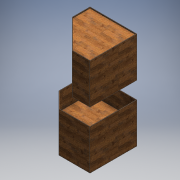
# Autodesk Inventor part: esquinero
Saved by Autodesk Inventor 2016 (Build 200138000, 138)
## iProperties
Created: 2015-11-25
Part Number: esquinero
Material: Generic
Document SubType Name: Modeling
Designer: Daniela
Density: 1 g/cm^3
Appearance: White
Author: Daniela
Autodesk Inventor part; units mm, degrees
ref_plane "YZ Plane" through (0, 0, 0) normal (1, 0, 0) x (0, 1, 0)
ref_plane "XZ Plane" through (0, 0, 0) normal (0, 1, 0) x (-1, 0, 0)
ref_plane "XY Plane" through (0, 0, 0) normal (0, 0, 1) x (1, 0, 0)
sketch "Sketch2" plane through (0, 0, 0) normal (0, 0, 1) x (1, 0, 0)
  line L0 (0, 0) -> (1050, 0) construction
  line L1 (1050, 0) -> (1050, 1050) construction
  line L2 (1050, 1050) -> (0, 1050) construction
  line L3 (0, 1050) -> (0, 0) construction
  line L4 (350, 0) -> (0, 350)
  line L5 (0, 350) -> (0, 1050)
  line L6 (0, 1050) -> (1050, 1050)
  line L7 (1050, 1050) -> (1050, 0)
  line L8 (1050, 0) -> (350, 0)
  dimension "d6" = 45
  dimension "profundidad" = 700
  dimension "d8" = 350
  constraints: 18 end point, 4 collinear, 2 parallel, 2 perpendicular, 2 point on line, 1 horizontal
  measures "d6" angle of L4 L0
  measures "profundidad" distance from line of L2 L4.end
  measures "d8" distance of L0.start L4.end
extrude "Extrusion1" add sketch "Sketch2" along normal blind 10
ref_plane "Work Plane1" through (0, 0, -80) normal (0, 0, -1) x (-1, 0, 0)
sketch "Sketch4" plane through (0, 0, -80) normal (0, 0, -1) x (-1, 0, 0)
  line L0 (-1050, 1050) -> (0, 1050) projected
  line L1 (-1050, 0) -> (-1050, 1050) projected
  line L2 (-350, 0) -> (-1050, 0) projected
  line L3 (0, 350) -> (-350, 0) projected
  line L4 (0, 1050) -> (0, 350) projected
  line L5 (-1040, 1040) -> (-10, 1040)
  line L6 (-10, 1040) -> (-10, 354.1421)
  line L7 (-10, 354.1421) -> (-354.1421, 10)
  line L8 (-354.1421, 10) -> (-1040, 10)
  line L9 (-1040, 10) -> (-1040, 1040)
  point P0 (0, 0)
  dimension "d12" = 10
  constraints: 10 end point, 4 other
  measures "d12" distance between parallel lines of L9 L1
extrude "Extrusion2" add sketch "Sketch4" against normal blind 900
sketch "Sketch5" plane through (350, 0, 820) normal (-0.7071068, -0.7071068, 0) x (-0.7071068, 0.7071068, 0)
  line L0 (0, 900) -> (0, 0) construction
  line L1 (494.9747, 900) -> (494.9747, 0) construction
  line L2 (494.9747, 0) -> (0, 0) construction
  line L3 (490.8326, 810) -> (4.1421, 810) construction
  line L4 (464.9747, 30) -> (34.1421, 30)
  line L5 (34.1421, 30) -> (34.1421, 810)
  line L6 (34.1421, 810) -> (464.9747, 810)
  line L7 (464.9747, 810) -> (464.9747, 30)
  line L8 (4.1421, 810) -> (4.1421, 0) projected
  point P0 (247.4874, 820)
  dimension "d15" = 30
  dimension "d16" = 30
  dimension "d17" = 30
  dimension "d18" = 0
  constraints: 8 end point, 2 parallel, 1 horizontal, 1 perpendicular
  measures "d15" distance between parallel lines of L2 L4
  measures "d16" distance between parallel lines of L1 L7
  measures "d17" distance between parallel lines of L8 L5
  measures "d18" distance between parallel lines of L3 L6
extrude "Extrusion3" cut sketch "Sketch5" against normal up to next
ref_plane "Work Plane2" through (0, 0, 1200) normal (0, 0, 1) x (1, 0, 0)
sketch "Sketch12" plane through (0, 0, 1200) normal (0, 0, 1) x (1, 0, 0)
  line L0 (1050, 1050) -> (0, 1050) projected
  line L1 (0, 1050) -> (0, 350) construction
  line L2 (0, 350) -> (350, 0) construction
  line L3 (350, 0) -> (1050, 0) construction
  line L4 (1050, 0) -> (1050, 1050) projected
  line L5 (0, 650) -> (650, 0)
  line L6 (0, 650) -> (0, 1050)
  line L7 (650, 0) -> (1050, 0)
  point P0 (0, 0)
  dimension "d32" = 400
  constraints: 6 end point, 2 collinear, 2 point on line, 1 parallel
  measures "d32" distance from line of L0 L5.start
extrude "Extrusion8" add sketch "Sketch12" along normal blind 10
sketch "Sketch13" plane through (0, 0, 1210) normal (0, 0, 1) x (1, 0, 0)
  line L0 (1050, 1050) -> (0, 1050) projected
  line L1 (0, 1050) -> (0, 650) projected
  line L2 (0, 650) -> (650, 0) projected
  line L3 (650, 0) -> (1050, 0) projected
  line L4 (1050, 0) -> (1050, 1050) projected
  line L5 (10, 1040) -> (1040, 1040)
  line L6 (1040, 1040) -> (1040, 10)
  line L7 (1040, 10) -> (654.1421, 10)
  line L8 (654.1421, 10) -> (10, 654.1421)
  line L9 (10, 654.1421) -> (10, 1040)
  point P0 (0, 0)
  dimension "d35" = 10
  constraints: 10 end point, 4 other
  measures "d35" distance between parallel lines of L5 L0
extrude "Extrusion9" add sketch "Sketch13" along normal blind 750
sketch "Sketch14" plane through (650, 0, 1960) normal (-0.7071068, -0.7071068, 0) x (-0.7071068, 0.7071068, 0)
  line L0 (915.0967, 750) -> (4.1421, 750) projected
  line L1 (915.0967, 750) -> (915.0967, 0) construction
  line L2 (4.1421, 750) -> (4.1421, 0) construction
  line L3 (915.0967, 30) -> (4.1421, 30)
  line L4 (915.0967, 750) -> (915.0967, 30)
  line L5 (4.1421, 30) -> (4.1421, 750)
  point P0 (459.6194, 1960)
  dimension "d38" = 30
  constraints: 6 end point, 2 perpendicular, 2 point on line, 1 collinear
  measures "d38" distance from line of L3 L1.end
extrude "Extrusion10" cut sketch "Sketch14" against normal up to next
sketch "Sketch15" plane through (647.0711, 2.9289, 1930) normal (0, 0, -1) x (-0.7071068, -0.7071068, 0)
  line L0 (-10, 0) -> (-10, 910.9545) projected
  line L1 (-282.8427, -272.8427) -> (-10, 0) projected
  line L2 (-1011.1627, 455.4773) -> (-282.8427, -272.8427) projected
  line L3 (-282.8427, 1183.7973) -> (-1011.1627, 455.4773) projected
  line L4 (-10, 910.9545) -> (-282.8427, 1183.7973) projected
  point P0 (459.6194, 455.4773)
  point P1 (0, 10)
  point P2 (0, 900.9545)
extrude "Extrusion11" add sketch "Sketch15" against normal blind 10
ref_plane "Work Plane3" through (1040, 1040, 1555) normal (0, 0, -1) x (-1, 0, 0)
ref_plane "Work Plane4" through (0, 0, 410) normal (0, 0, 1) x (1, 0, 0)
sketch "Sketch16" plane through (1040, 1040, 1555) normal (0, 0, -1) x (-1, 0, 0)
  line L0 (385.8579, -1030) -> (1030, -385.8579) construction
  line L1 (1030, 0) -> (1030, -685.8579) construction
  line L2 (0, 0) -> (1030, 0) construction
  line L3 (0, -1030) -> (0, 0) construction
  line L4 (685.8579, -1030) -> (0, -1030) construction
  line L5 (0, 0) -> (0, -1030) construction
  line L6 (0, -1030) -> (685.8579, -1030) construction
  line L7 (685.8579, -1030) -> (1030, -685.8579) construction
  line L8 (1030, -685.8579) -> (1030, 0) construction
  line L9 (1030, 0) -> (0, 0) construction
  line L10 (385.8579, -1030) -> (1030, -385.8579) projected
  line L11 (1030, -385.8579) -> (1030, 0) projected
  line L12 (1030, -385.8579) -> (1030, 0)
  line L13 (0, 0) -> (1030, 0) projected
  line L14 (1030, 0) -> (0, 0)
  line L15 (-10, -1040) -> (-10, 10) projected
  line L16 (0, 0) -> (0, -1030) projected
  line L17 (0, 0) -> (0, -1030)
  line L18 (0, -1030) -> (385.8579, -1030)
  point P0 (1040, -1040)
  point P1 (0, 0)
  point P2 (-644.1421, 0)
  point P3 (-1030, 385.8579)
  point P4 (-385.8579, 1030)
  point P5 (0, 644.1421)
  constraints: 8 end point, 3 perpendicular, 1 collinear, 2 other
extrude "Extrusion12" add sketch "Sketch16" along normal blind 10
sketch "Sketch17" plane through (0, 0, 410) normal (0, 0, 1) x (1, 0, 0)
  line L0 (1040, 1040) -> (1040, 10) projected
  line L1 (1040, 10) -> (354.1421, 10) projected
  line L2 (354.1421, 10) -> (10, 354.1421) projected
  line L3 (10, 354.1421) -> (10, 1040) projected
  line L4 (10, 1040) -> (1040, 1040) projected
  point P0 (0, 0)
extrude "Extrusion13" add sketch "Sketch17" along normal blind 10
equation "\"d8\" = 0.5 * profundidad"
equation "\"d12\" = espesor"
equation "\"d15\" = 3 * espesor"
equation "\"d16\" = 3 * espesor"
equation "\"d17\" = 3 * espesor"
equation "\"d33\" = espesor"
equation "\"d35\" = espesor"
equation "\"d38\" = 3 * espesor"
equation "\"d41\" = espesor"
equation "\"d45\" = espesor"
equation "\"d47\" = espesor"
equation "\"d43\" = 0.5 * h_sup"
equation "\"espesor\" = 10"
equation "\"h_sup\" = 750"
body "Solid1"
